Autodesk Inventor part; units mm, degrees
(part 2 of 2)
sketch "草圖10" plane through (0, -6, 0) normal (0, -1, 0) x (1, 0, 0)
  circle A0 centre (0, 0) radius 11
  line L0 (-11.5, -1) -> (-10.5, -1)
  line L1 (-10.5, -1) -> (-10.5, 1)
  line L2 (-10.5, 1) -> (-11.5, 1)
  line L3 (-11.5, 1) -> (-11.5, -1)
  line L4 (-11.5, -1) -> (-10.5, 1) construction
  line L5 (-10.5, -1) -> (-11.5, 1) construction
  line L6 (-10.4785, -1.2049) -> (-11.4566, -1.4128)
  line L7 (-11.4566, -1.4128) -> (-11.0408, -3.3691)
  line L8 (-10.0626, -3.1612) -> (-10.4785, -1.2049)
  line L9 (-11.0408, -3.3691) -> (-10.0626, -3.1612)
  line L10 (-9.999, -3.3572) -> (-10.9125, -3.7639)
  line L11 (-10.9125, -3.7639) -> (-10.099, -5.591)
  line L12 (-9.1855, -5.1843) -> (-9.999, -3.3572)
  line L13 (-10.099, -5.591) -> (-9.1855, -5.1843)
  line L14 (-9.0825, -5.3627) -> (-9.8915, -5.9505)
  line L15 (-9.8915, -5.9505) -> (-8.7159, -7.5685)
  line L16 (-7.9069, -6.9808) -> (-9.0825, -5.3627)
  line L17 (-8.7159, -7.5685) -> (-7.9069, -6.9808)
  line L18 (-7.769, -7.1339) -> (-8.4381, -7.877)
  line L19 (-8.4381, -7.877) -> (-6.9519, -9.2153)
  line L20 (-6.2827, -8.4722) -> (-7.769, -7.1339)
  line L21 (-6.9519, -9.2153) -> (-6.2827, -8.4722)
  line L22 (-6.116, -8.5933) -> (-6.616, -9.4593)
  line L23 (-6.616, -9.4593) -> (-4.884, -10.4593)
  line L24 (-4.384, -9.5933) -> (-6.116, -8.5933)
  line L25 (-4.884, -10.4593) -> (-4.384, -9.5933)
  line L26 (-4.1957, -9.6771) -> (-4.5048, -10.6281)
  line L27 (-4.5048, -10.6281) -> (-2.6026, -11.2462)
  line L28 (-2.2936, -10.2951) -> (-4.1957, -9.6771)
  line L29 (-2.6026, -11.2462) -> (-2.2936, -10.2951)
  line L30 (-2.0921, -10.338) -> (-2.1966, -11.3325)
  line L31 (-2.1966, -11.3325) -> (-0.2076, -11.5415)
  line L32 (-0.103, -10.547) -> (-2.0921, -10.338)
  line L33 (-0.2076, -11.5415) -> (-0.103, -10.547)
  line L34 (0.103, -10.547) -> (0.2076, -11.5415)
  line L35 (0.2076, -11.5415) -> (2.1966, -11.3325)
  line L36 (2.0921, -10.338) -> (0.103, -10.547)
  line L37 (2.1966, -11.3325) -> (2.0921, -10.338)
  line L38 (2.2936, -10.2951) -> (2.6026, -11.2462)
  line L39 (2.6026, -11.2462) -> (4.5048, -10.6281)
  line L40 (4.1957, -9.6771) -> (2.2936, -10.2951)
  line L41 (4.5048, -10.6281) -> (4.1957, -9.6771)
  line L42 (4.384, -9.5933) -> (4.884, -10.4593)
  line L43 (4.884, -10.4593) -> (6.616, -9.4593)
  line L44 (6.116, -8.5933) -> (4.384, -9.5933)
  line L45 (6.616, -9.4593) -> (6.116, -8.5933)
  line L46 (6.2827, -8.4722) -> (6.9519, -9.2153)
  line L47 (6.9519, -9.2153) -> (8.4381, -7.877)
  line L48 (7.769, -7.1339) -> (6.2827, -8.4722)
  line L49 (8.4381, -7.877) -> (7.769, -7.1339)
  line L50 (7.9069, -6.9808) -> (8.7159, -7.5685)
  line L51 (8.7159, -7.5685) -> (9.8915, -5.9505)
  line L52 (9.0825, -5.3627) -> (7.9069, -6.9808)
  line L53 (9.8915, -5.9505) -> (9.0825, -5.3627)
  line L54 (9.1855, -5.1843) -> (10.099, -5.591)
  line L55 (10.099, -5.591) -> (10.9125, -3.7639)
  line L56 (9.999, -3.3572) -> (9.1855, -5.1843)
  line L57 (10.9125, -3.7639) -> (9.999, -3.3572)
  line L58 (10.0626, -3.1612) -> (11.0408, -3.3691)
  line L59 (11.0408, -3.3691) -> (11.4566, -1.4128)
  line L60 (10.4785, -1.2049) -> (10.0626, -3.1612)
  line L61 (11.4566, -1.4128) -> (10.4785, -1.2049)
  line L62 (10.5, -1) -> (11.5, -1)
  line L63 (11.5, -1) -> (11.5, 1)
  line L64 (10.5, 1) -> (10.5, -1)
  line L65 (11.5, 1) -> (10.5, 1)
  line L66 (10.4785, 1.2049) -> (11.4566, 1.4128)
  line L67 (11.4566, 1.4128) -> (11.0408, 3.3691)
  line L68 (10.0626, 3.1612) -> (10.4785, 1.2049)
  line L69 (11.0408, 3.3691) -> (10.0626, 3.1612)
  line L70 (9.999, 3.3572) -> (10.9125, 3.7639)
  line L71 (10.9125, 3.7639) -> (10.099, 5.591)
  line L72 (9.1855, 5.1843) -> (9.999, 3.3572)
  line L73 (10.099, 5.591) -> (9.1855, 5.1843)
  line L74 (9.0825, 5.3627) -> (9.8915, 5.9505)
  line L75 (9.8915, 5.9505) -> (8.7159, 7.5685)
  line L76 (7.9069, 6.9808) -> (9.0825, 5.3627)
  line L77 (8.7159, 7.5685) -> (7.9069, 6.9808)
  line L78 (7.769, 7.1339) -> (8.4381, 7.877)
  line L79 (8.4381, 7.877) -> (6.9519, 9.2153)
  line L80 (6.2827, 8.4722) -> (7.769, 7.1339)
  line L81 (6.9519, 9.2153) -> (6.2827, 8.4722)
  line L82 (6.116, 8.5933) -> (6.616, 9.4593)
  line L83 (6.616, 9.4593) -> (4.884, 10.4593)
  line L84 (4.384, 9.5933) -> (6.116, 8.5933)
  line L85 (4.884, 10.4593) -> (4.384, 9.5933)
  line L86 (4.1957, 9.6771) -> (4.5048, 10.6281)
  line L87 (4.5048, 10.6281) -> (2.6026, 11.2462)
  line L88 (2.2936, 10.2951) -> (4.1957, 9.6771)
  line L89 (2.6026, 11.2462) -> (2.2936, 10.2951)
  line L90 (2.0921, 10.338) -> (2.1966, 11.3325)
  line L91 (2.1966, 11.3325) -> (0.2076, 11.5415)
  line L92 (0.103, 10.547) -> (2.0921, 10.338)
  line L93 (0.2076, 11.5415) -> (0.103, 10.547)
  line L94 (-0.103, 10.547) -> (-0.2076, 11.5415)
  line L95 (-0.2076, 11.5415) -> (-2.1966, 11.3325)
  line L96 (-2.0921, 10.338) -> (-0.103, 10.547)
  line L97 (-2.1966, 11.3325) -> (-2.0921, 10.338)
  line L98 (-2.2936, 10.2951) -> (-2.6026, 11.2462)
  line L99 (-2.6026, 11.2462) -> (-4.5048, 10.6281)
  line L100 (-4.1957, 9.6771) -> (-2.2936, 10.2951)
  line L101 (-4.5048, 10.6281) -> (-4.1957, 9.6771)
  line L102 (-4.384, 9.5933) -> (-4.884, 10.4593)
  line L103 (-4.884, 10.4593) -> (-6.616, 9.4593)
  line L104 (-6.116, 8.5933) -> (-4.384, 9.5933)
  line L105 (-6.616, 9.4593) -> (-6.116, 8.5933)
  line L106 (-6.2827, 8.4722) -> (-6.9519, 9.2153)
  line L107 (-6.9519, 9.2153) -> (-8.4381, 7.877)
  line L108 (-7.769, 7.1339) -> (-6.2827, 8.4722)
  line L109 (-8.4381, 7.877) -> (-7.769, 7.1339)
  line L110 (-7.9069, 6.9808) -> (-8.7159, 7.5685)
  line L111 (-8.7159, 7.5685) -> (-9.8915, 5.9505)
  line L112 (-9.0825, 5.3627) -> (-7.9069, 6.9808)
  line L113 (-9.8915, 5.9505) -> (-9.0825, 5.3627)
  line L114 (-9.1855, 5.1843) -> (-10.099, 5.591)
  line L115 (-10.099, 5.591) -> (-10.9125, 3.7639)
  line L116 (-9.999, 3.3572) -> (-9.1855, 5.1843)
  line L117 (-10.9125, 3.7639) -> (-9.999, 3.3572)
  line L118 (-10.0626, 3.1612) -> (-11.0408, 3.3691)
  line L119 (-11.0408, 3.3691) -> (-11.4566, 1.4128)
  line L120 (-10.4785, 1.2049) -> (-10.0626, 3.1612)
  line L121 (-11.4566, 1.4128) -> (-10.4785, 1.2049)
  point P0 (-11, 0)
  dimension "d65" = 22
  dimension "d66" = 1
  dimension "d67" = 2
  dimension "d70" = 360
  constraints: 244 end point, 2 midpoint, 2 parallel, 1 coincident, 1 horizontal, 1 horizontal alignment, 1 perpendicular, 243 other
  measures "d66" distance of L2.end L1.end
  measures "d67" distance of L1.end L0.end
extrude "擠出10" add sketch "草圖10" along normal blind 1 contours A0 L62 L64 L65 | A0 L65 L63 L62 | L66 L68 L69 A0 | A0 L69 L67 L66 | L61 L59 L58 A0 | A0 L58 L60 L61 | L70 L72 L73 A0 | A0 L73 L71 L70 | L57 L55 L54 A0 | A0 L54 L56 L57 | L74 L76 L77 A0 | A0 L77 L75 L74 | L53 L51 L50 A0 | A0 L50 L52 L53 | L78 L80 L81 A0 | A0 L81 L79 L78 | L49 L47 L46 A0 | A0 L46 L48 L49 | L82 L84 L85 A0 | A0 L85 L83 L82 | L45 L43 L42 A0 | A0 L42 L44 L45 | L86 L88 L89 A0 | A0 L89 L87 L86 | L41 L39 L38 A0 | A0 L38 L40 L41 | L90 L92 L93 A0 | A0 L93 L91 L90 | L37 L35 L34 A0 | A0 L34 L36 L37 | L94 L96 L97 A0 | A0 L97 L95 L94 | L33 L31 L30 A0 | A0 L30 L32 L33 | L98 L100 L101 A0 | A0 L101 L99 L98 | L29 L27 L26 A0 | A0 L26 L28 L29 | L102 L104 L105 A0 | A0 L105 L103 L102 | L25 L23 L22 A0 | A0 L22 L24 L25 | L106 L108 L109 A0 | A0 L109 L107 L106 | L21 L19 L18 A0 | A0 L18 L20 L21 | L110 L112 L113 A0 | A0 L113 L111 L110 | L17 L15 L14 A0 | A0 L14 L16 L17 | L114 L116 L117 A0 | A0 L117 L115 L114 | L13 L11 L10 A0 | A0 L10 L12 L13 | L118 L120 L121 A0 | A0 L121 L119 L118 | L9 L7 L6 A0 | A0 L6 L8 L9 | L2 L1 L0 A0 | A0 L0 L3 L2
pattern_linear "矩形陣列1" count 2 spacing 2 along (0, -1, 0) of "擠出10", "擠出9"
sketch "草圖11" plane through (2.2936, -9, 10.2951) normal (0, -1, 0) x (0.9510565, 0, -0.309017)
  circle A0 centre (1, -10.5) radius 11
  line L0 (-10, -10.5) -> (12, -10.5)
  dimension "d77" = 22
  constraints: 2 end point, 2 point on circle, 1 centre point, 1 coincident, 1 horizontal
  measures "d77" diameter of A0
revolve "迴轉1" add sketch "草圖11" angle 180 about axis through (-10.4616, -9, 3.3992) along (0.9510565, 0, -0.309017) picked at (-2.6667, -7.092) contours L0 A0
sketch "草圖12" plane through (0, 0, 0) normal (1, 0, 0) x (0, 1, 0)
  arc A0 (-9, 11) -> (-9, -11) centre (-9, 0) ccw projected
  arc A1 (-9, 11) -> (-9, -11) centre (-9, 0) ccw
  arc A2 (-8.4507, 9.9849) -> (-8.4507, -9.9849) centre (-9, 0) ccw
  line L0 (-8, 11.2462) -> (-9, 11.2462) projected
  line L1 (-8, 6.9808) -> (-8, 6.6169) projected
  line L2 (-9, -11) -> (-9, -10)
  line L3 (-9, 11) -> (-9, 10)
  line L4 (-8, 10.4785) -> (-8, 11.4158) projected
  point P0 (0, 0)
  dimension "d79" = 1
  constraints: 8 point on circle, 4 end point, 2 centre point, 1 concentric, 1 parallel
  measures "d79" radial gap between concentric circles of A0 A2
extrude "擠出11" cut sketch "草圖12" along normal mid plane 1
sketch "草圖13" plane through (0, 0, 0) normal (0, 0, 1) x (1, 0, 0)
  arc A0 (-11, -9) -> (-0.5, -19.9886) centre (0, -9) ccw projected
  arc A1 (0.5, -19.9886) -> (11, -9) centre (0, -9) ccw projected
  arc A2 (-11, -9) -> (11, -9) centre (0, -9) ccw
  arc A3 (-10, -9) -> (10, -9) centre (0, -9) ccw
  line L0 (11, -9) -> (10.9545, -9) projected
  line L1 (-11, -9) -> (11, -9)
  point P0 (0, 0)
  point P1 (-0.5, -19.9886)
  dimension "d82" = 1
  constraints: 6 point on circle, 2 centre point, 2 concentric, 2 end point, 2 point on line, 1 horizontal
  measures "d82" radial gap between concentric circles of A1 A3
extrude "擠出12" cut sketch "草圖13" along normal mid plane 1 contours L1 A3 L0 A1 A2 A0
